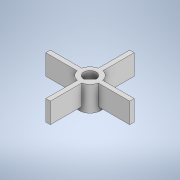
# Autodesk Inventor part: wheel of the walls
Saved by Autodesk Inventor 2022 (Build 260153000, 153)
## iProperties
Created: 2022-03-03
Part Number: wheel of the walls
Material: Generic
Document SubType Name: Modeling
Designer: Alicia
Density: 1 g/cm^3
Appearance: Default
Author: Alicia
Autodesk Inventor part; units mm, degrees
ref_plane "YZ Plane" through (0, 0, 0) normal (1, 0, 0) x (0, 1, 0)
ref_plane "XZ Plane" through (0, 0, 0) normal (0, 1, 0) x (-1, 0, 0)
ref_plane "XY Plane" through (0, 0, 0) normal (0, 0, 1) x (1, 0, 0)
sketch "Sketch1" plane through (0, 0, 0) normal (0, 1, 0) x (-1, 0, 0)
  line L0 (1, -18.473) -> (1, -4.6435)
  line L1 (1, 4.6435) -> (1, 18.473)
  line L2 (-1, -18.473) -> (-1, -4.6435)
  line L3 (-1, 4.6435) -> (-1, 18.473)
  line L4 (18.473, 1) -> (4.6435, 1)
  line L5 (-4.6435, 1) -> (-18.473, 1)
  line L6 (18.473, -1) -> (4.6435, -1)
  line L7 (-4.6435, -1) -> (-18.473, -1)
  arc A0 (-18.473, 1) -> (-18.473, -1) centre (0, 0) ccw
  arc A1 (-1, -18.473) -> (1, -18.473) centre (0, 0) ccw
  arc A2 (18.473, -1) -> (18.473, 1) centre (0, 0) ccw
  arc A3 (1, 18.473) -> (-1, 18.473) centre (0, 0) ccw
  arc A4 (4.6435, 1) -> (1, 4.6435) centre (0, 0) ccw
  arc A5 (-1, 4.6435) -> (-4.6435, 1) centre (0, 0) ccw
  arc A6 (-4.6435, -1) -> (-1, -4.6435) centre (0, 0) ccw
  arc A7 (1, -4.6435) -> (4.6435, -1) centre (0, 0) ccw
  point P0 (1, -4.899)
  point P1 (1, 4.899)
  point P2 (4.899, -1)
  point P3 (-1, 4.899)
  point P4 (4.899, 1)
  point P5 (-4.899, 1)
  point P6 (-4.899, -1)
  point P7 (-1, -4.899)
  point P8 (-18.9737, -1)
  point P9 (-1, -18.9737)
  point P10 (1, -18.9737)
  point P11 (18.9737, -1)
  point P12 (18.9737, 1)
  point P13 (1, 18.9737)
  point P14 (-1, 18.9737)
  point P15 (-18.9737, 1)
  point P16 (17.4714, 1)
  point P17 (1, 17.4714)
  point P18 (-1, 17.4714)
  point P19 (-17.4714, 1)
  point P20 (-17.4714, -1)
  point P21 (-1, -17.4714)
  point P22 (1, -17.4714)
  point P23 (17.4714, -1)
  constraints: 24 point on line, 16 end point, 16 point on circle, 8 centre point, 1 coincident
extrude "Extrusion1" add sketch "Sketch1" along normal blind 9
sketch "Sketch2" plane through (0, 0, 0) normal (0, -1, 0) x (1, 0, 0)
  circle A0 centre (0, 0) radius 4.75
  dimension "d11" = 9.5
  constraints: 1 centre point
  measures "d11" diameter of A0
extrude "Extrusion2" add sketch "Sketch2" along normal blind 2
sketch "Sketch3" plane through (0, 9, 0) normal (0, 1, 0) x (1, 0, 0)
  arc A0 (2.75, 0) -> (0, -2.75) centre (0, 0) ccw
  line L0 (0, -2.75) -> (2.75, 0)
  dimension "d6" = 5.5
  constraints: 2 end point, 2 point on circle, 1 centre point, 1 coincident
  measures "d6" diameter of A0
extrude "Extrusion3" cut sketch "Sketch3" against normal through all
body "Solid1"
